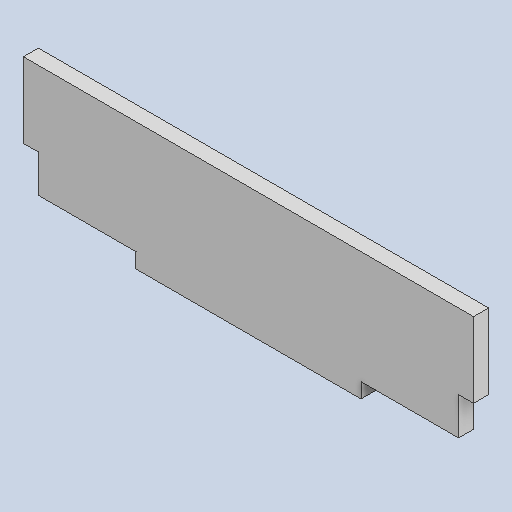
# Autodesk Inventor part: bottom_hinge_002
Saved by Autodesk Inventor 2025.2 (Build 292293000, 293)
## iProperties
Created: 2025-03-24
Part Number: bottom_hinge_002
Material: Generic
Document SubType Name: Sheet Metal
Designer: Caspe
Density: 1 g/cm^3
Sheet Metal Rule: Default_mm
Appearance: Default
Author: Caspe
Autodesk Inventor part; units mm, degrees
ref_plane "YZ Plane" through (0, 0, 0) normal (1, 0, 0) x (0, 1, 0)
ref_plane "XZ Plane" through (0, 0, 0) normal (0, 1, 0) x (-1, 0, 0)
ref_plane "XY Plane" through (0, 0, 0) normal (0, 0, 1) x (1, 0, 0)
sketch "Sketch1" plane through (0, 0, 0) normal (0, 0, 1) x (1, 0, 0)
  line L0 (0, 0) -> (56, 0)
  line L1 (56, 0) -> (56, 15)
  line L2 (56, 15) -> (0, 15)
  line L3 (0, 15) -> (0, 0)
  line L4 (13, 0) -> (43, 0)
  line L5 (43, 0) -> (43, -2)
  line L6 (43, -2) -> (13, -2)
  line L7 (13, -2) -> (13, 0)
  line L8 (0, 5) -> (-2, 5)
  line L9 (-2, 5) -> (-2, 15)
  line L10 (-2, 15) -> (0, 15)
  line L11 (0, 15) -> (0, 5)
  line L12 (28, 15) -> (28, 0)
  line L13 (56, 5) -> (58, 5)
  line L14 (58, 5) -> (58, 15)
  line L15 (58, 15) -> (56, 15)
  point P0 (0, 15)
  dimension "d0" = 56
  dimension "d1" = 30
  dimension "d2" = 2
  dimension "d3" = 15
  dimension "d4" = 2
  dimension "d5" = 10
  dimension "d6" = 5
  measures "d0" distance of L2.end L1.end
  measures "d1" distance of L5.end L6.end
  measures "d2" distance of L4.end L5.end
  measures "d3" distance between parallel lines of L2 L0
  measures "d4" distance of L9.end L10.end
  measures "d5" distance of L8.end L9.end
  measures "d6" distance between parallel lines of L0 L8
extrude "Plate1" add sketch "Sketch1" along normal blind 2
equation "\"d0\" = A_width + 2 * A_joint_tolerance"
equation "\"d2\" = plate_thickness"
equation "\"d4\" = plate_thickness"
equation "\"d7\" = Thickness"
equation "\"Thickness\" = plate_thickness"
equation "\"BendRadius\" = Thickness"
equation "\"BendReliefWidth\" = Thickness"
equation "\"BendReliefDepth\" = 0.5 * Thickness"
equation "\"CornerReliefSize\" = 4 * Thickness"
equation "\"MinimumRemnant\" = 2 * Thickness"
equation "\"TransitionRadius\" = BendRadius"
equation "\"JacobiRadiusSize\" = BendRadius"
equation "\"GapSize\" = Thickness"
equation "\"l___________\" = 0"
equation "\"l__________\" = 0"
equation "\"l_________\" = 0"
equation "\"rivet_diameter\" = 3.35"
equation "\"plate_thickness\" = 2"
equation "\"l________\" = 0"
equation "\"A_joint_tolerance\" = 3"
equation "\"A_B_spacing\" = 2"
equation "\"L_Piston_Bottom\" = 21"
equation "\"L_Piston_Top\" = 25"
equation "\"A_width\" = 50"
body "Solid1"
